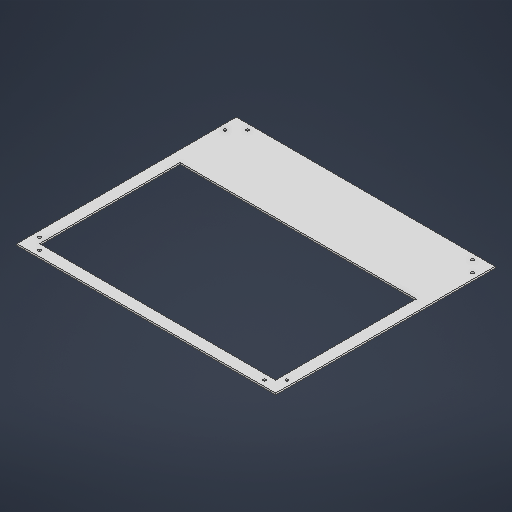
# Autodesk Inventor part: TapaFrontal
Saved by Autodesk Inventor 2026.2 (Build 302298010, 298A)
## iProperties
Created: 2026-04-14
Part Number: TapaFrontal
Material: Generic
Document SubType Name: Modeling
Designer: grego
Density: 1 g/cm^3
Appearance: Default
Author: grego
Autodesk Inventor part; units mm, degrees
ref_plane "YZ Plane" through (0, 0, 0) normal (1, 0, 0) x (0, 1, 0)
ref_plane "XZ Plane" through (0, 0, 0) normal (0, 1, 0) x (-1, 0, 0)
ref_plane "XY Plane" through (0, 0, 0) normal (0, 0, 1) x (1, 0, 0)
sketch "Sketch1" plane through (0, 0, 0) normal (0, 1, 0) x (-1, 0, 0)
  line L0 (-230, 195) -> (230, 195)
  line L1 (230, 195) -> (230, -195)
  line L2 (230, -195) -> (-230, -195)
  line L3 (-230, -195) -> (-230, 195)
  line L4 (-230, 195) -> (230, -195) construction
  line L5 (230, 195) -> (-230, -195) construction
  line L6 (210, -75) -> (210, 175)
  line L7 (210, 175) -> (-210, 175)
  line L8 (-210, 175) -> (-210, -75)
  line L9 (230, -195) -> (200, -195)
  line L10 (230, -195) -> (230, -165)
  line L11 (0, 0) -> (0, -25.7255)
  line L12 (0, 0) -> (16.1441, 0)
  circle A0 centre (200, -185) radius 2.5
  circle A1 centre (220, -165) radius 2.5
  circle A2 centre (-200, -185) radius 2.5
  circle A3 centre (-220, -165) radius 2.5
  circle A4 centre (200, 185) radius 2.5
  circle A5 centre (220, 165) radius 2.5
  circle A6 centre (-220, 165) radius 2.5
  circle A7 centre (-200, 185) radius 2.5
  line L13 (-210, 175) -> (-210, -75)
  line L14 (-210, -75) -> (210, -75)
  line L15 (206.4103, -175) -> (210, -175)
  dimension "d0" = 460
  dimension "d1" = 390
  dimension "d6" = 30
  dimension "d10" = 250
  constraints: 32 end point, 8 centre point, 6 symmetric about line, 4 parallel, 3 perpendicular, 3 point on line, 2 horizontal, 2 midpoint, 1 vertical, 6 other
  measures "d0" distance of L1.end L2.end
  measures "d1" distance of L0.end L1.end
  measures "d6" distance of L1.end L9.end
  measures "d10" distance of L8.end L7.end
extrude "Extrusion1" add sketch "Sketch1" along normal blind 3
body "Solid1"
